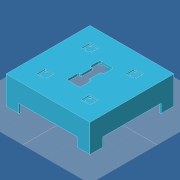
# Autodesk Inventor part: Sensorlamp_Cover
Saved by Autodesk Inventor 2016 SP2 (Build 200236200, 236)
## iProperties
Created: 2017-11-14
Part Number: Sensorlamp_Cover
Material: Generisch
Document SubType Name: Modeling
Designer: User
Density: 1 g/cm^3
Appearance: Türkis
Author: User
Autodesk Inventor part; units mm, degrees
ref_plane "YZ Plane" through (0, 0, 0) normal (1, 0, 0) x (0, 1, 0)
ref_plane "XZ Plane" through (0, 0, 0) normal (0, 1, 0) x (-1, 0, 0)
ref_plane "XY Plane" through (0, 0, 0) normal (0, 0, 1) x (1, 0, 0)
sketch "LED" plane through (0, 0, 0) normal (0, 0, 1) x (1, 0, 0)
  line L0 (-24, 24) -> (-16, 24)
  line L1 (-16, 24) -> (-16, 16)
  line L2 (-16, 16) -> (-24, 16)
  line L3 (-24, 16) -> (-24, 24)
  line L4 (-24, 24) -> (-16, 16) construction
  line L5 (-16, 24) -> (-24, 16) construction
  circle A0 centre (-22.5, 22.5) radius 1
  circle A1 centre (-17.5, 22.5) radius 1
  circle A2 centre (-22.5, 17.5) radius 1
  circle A3 centre (-17.5, 17.5) radius 1
  point P0 (-20, 20)
  point P1 (-20, 20)
  point P2 (-20, 20)
  point P3 (-20, 20)
  dimension "d11" = 8
  dimension "d12" = 8
  dimension "d20" = 2
  dimension "d21" = 5
  dimension "d22" = 5
  measures "d11" distance of L1.end L2.end
  measures "d12" distance of L0.end L1.end
  measures "d20" diameter of A0
  measures "d21" distance of A1.centre A0.centre
  measures "d22" distance of A2.centre A0.centre
sketch "Skizze1" plane through (0, 0, 0) normal (0, 0, 1) x (1, 0, 0)
  line L0 (-37.5, -37.5) -> (37.5, -37.5)
  line L1 (37.5, -37.5) -> (37.5, 37.5)
  line L2 (37.5, 37.5) -> (-37.5, 37.5)
  line L3 (-37.5, 37.5) -> (-37.5, -37.5)
  line L4 (-37.5, -37.5) -> (37.5, 37.5) construction
  line L5 (37.5, -37.5) -> (-37.5, 37.5) construction
  line L6 (-5, 15) -> (5, 15)
  line L7 (6, 14) -> (6, 6.75)
  line L8 (5, 5.75) -> (3.75, 5.75)
  line L9 (3.75, 5.75) -> (3.75, -4.25)
  line L10 (3.75, -4.25) -> (5, -4.25)
  line L11 (6, -5.25) -> (6, -14)
  line L12 (5, -15) -> (-5, -15)
  line L13 (-6, -14) -> (-6, -5.25)
  line L14 (-5, -4.25) -> (-3.75, -4.25)
  line L15 (-3.75, -4.25) -> (-3.75, 5.75)
  line L16 (-3.75, 5.75) -> (-5, 5.75)
  line L17 (-6, 6.75) -> (-6, 14)
  arc A0 (-5, 15) -> (-6, 14) centre (-5, 14) ccw
  arc A1 (6, 14) -> (5, 15) centre (5, 14) ccw
  arc A2 (-6, -14) -> (-5, -15) centre (-5, -14) ccw
  arc A3 (5, -15) -> (6, -14) centre (5, -14) ccw
  arc A4 (6, -5.25) -> (5, -4.25) centre (5, -5.25) ccw
  arc A5 (-5, -4.25) -> (-6, -5.25) centre (-5, -5.25) ccw
  arc A6 (-6, 6.75) -> (-5, 5.75) centre (-5, 6.75) ccw
  arc A7 (5, 5.75) -> (6, 6.75) centre (5, 6.75) ccw
  line L18 (0, 15) -> (0, -15) construction
  line L19 (-52.5, 0) -> (52.5, 0) projected
  line L20 (0, -52.5) -> (0, 52.5) projected
  circle A8 centre (0, -18.5) radius 3.5
  circle A9 centre (0, 18.5) radius 3.5
  line L21 (3.5, -18.5) -> (3.5, -15)
  line L22 (-3.5, -18.5) -> (-3.5, -15)
  line L23 (-3.5, 18.5) -> (-3.5, 15)
  line L24 (3.5, 18.5) -> (3.5, 15)
  circle A10 centre (0, 18.5) radius 1.25
  circle A11 centre (0, -18.5) radius 1.25
  line L25 (-24, 24) -> (-16, 24)
  line L26 (-16, 24) -> (-16, 16)
  line L27 (-16, 16) -> (-24, 16)
  line L28 (-24, 16) -> (-24, 24)
  line L29 (-24, 24) -> (-16, 16) construction
  line L30 (-16, 24) -> (-24, 16) construction
  circle A12 centre (-22.5, 22.5) radius 1
  circle A13 centre (-17.5, 22.5) radius 1
  circle A14 centre (-22.5, 17.5) radius 1
  circle A15 centre (-17.5, 17.5) radius 1
  line L31 (16, 24) -> (24, 24)
  line L32 (24, 24) -> (24, 16)
  line L33 (24, 16) -> (16, 16)
  line L34 (16, 16) -> (16, 24)
  line L35 (16, 24) -> (24, 16) construction
  line L36 (24, 24) -> (16, 16) construction
  circle A16 centre (17.5, 22.5) radius 1
  circle A17 centre (22.5, 22.5) radius 1
  circle A18 centre (17.5, 17.5) radius 1
  circle A19 centre (22.5, 17.5) radius 1
  line L37 (16, -16) -> (24, -16)
  line L38 (24, -16) -> (24, -24)
  line L39 (24, -24) -> (16, -24)
  line L40 (16, -24) -> (16, -16)
  line L41 (16, -16) -> (24, -24) construction
  line L42 (24, -16) -> (16, -24) construction
  circle A20 centre (17.5, -17.5) radius 1
  circle A21 centre (22.5, -17.5) radius 1
  circle A22 centre (17.5, -22.5) radius 1
  circle A23 centre (22.5, -22.5) radius 1
  line L43 (-24, -16) -> (-16, -16)
  line L44 (-16, -16) -> (-16, -24)
  line L45 (-16, -24) -> (-24, -24)
  line L46 (-24, -24) -> (-24, -16)
  line L47 (-24, -16) -> (-16, -24) construction
  line L48 (-16, -16) -> (-24, -24) construction
  circle A24 centre (-22.5, -17.5) radius 1
  circle A25 centre (-17.5, -17.5) radius 1
  circle A26 centre (-22.5, -22.5) radius 1
  circle A27 centre (-17.5, -22.5) radius 1
  point P0 (0, 0)
  point P1 (6, -4.25)
  point P2 (6, -15)
  point P3 (-6, -4.25)
  point P4 (-6, 5.75)
  point P5 (0, 0)
  dimension "d23" = 40
  dimension "d24" = 40
  dimension "d0" = 75
  dimension "d1" = 75
  dimension "d2" = 30
  dimension "d3" = 12
  dimension "d5" = 7.5
  dimension "d6" = 9.25
  dimension "d8" = 10.75
  dimension "d9" = 10
  dimension "d10" = 1
  dimension "d34" = 2.5
  dimension "d37" = 37
  constraints: 46 end point, 22 point on line, 21 tangent, 20 point on circle, 12 centre point, 12 perpendicular, 9 equal radius, 6 midpoint, 3 horizontal, 2 coincident, 2 collinear, 2 parallel, 1 vertical
  measures "d0" distance of L2.end L1.end
  measures "d1" distance of L1.end L0.end
  measures "d2" distance between parallel lines of L12 L6
  measures "d3" distance between parallel lines of L7 L17
  measures "d5" distance between parallel lines of L9 L15
  measures "d6" distance between parallel lines of L16 L6
  measures "d8" distance between parallel lines of L12 L14
  measures "d9" distance between parallel lines of L14 L16
  measures "d10" radius of A0
  measures "d34" diameter of A10
  measures "d37" distance of A11.centre A9.centre
extrude "Extrusion1" add sketch "Skizze1" against normal blind 2 contours L3 L19 L15 L14 A5 L13 A2 L12 L22 A8 L20 L0 | L20 A8 L21 L12 A3 L11 A4 L10 L9 L19 L1 L0 | L3 L2 L20 A9 L23 L6 A0 L17 A6 L16 L15 L19 | A8 L20 A11 | L20 A11 A8 | L19 L9 L8 A7 L7 A1 L6 L24 A9 L20 L2 L1 | A11 L20 | L20 A11 | L22 L12 A8 | A8 L12 L21 | A9 L20 A10 | L20 A10 A9 | A9 L24 L6 | L6 L23 A9 | A10 L20 | L20 A10 | L25 L26 L27 L28 | L31 L32 L33 L34 | L37 L38 L39 L40 | L43 L44 L45 L46
extrude "Extrusion2" cut sketch "Skizze1" against normal blind 1 contours L25 L26 L27 L28 | L31 L32 L33 L34 | L37 L38 L39 L40 | L43 L44 L45 L46
sketch "Skizze2" plane through (0, 0, -2) normal (0, 0, -1) x (-1, 0, 0)
  line L0 (0, -52.5) -> (0, 52.5) projected
  circle A0 centre (22.5, -17.5) radius 1 projected
  circle A1 centre (17.5, -22.5) radius 1 projected
  circle A2 centre (22.5, -22.5) radius 1 projected
  circle A3 centre (17.5, -17.5) radius 1 projected
  circle A4 centre (-17.5, -17.5) radius 1 projected
  circle A5 centre (-22.5, -22.5) radius 1 projected
  circle A6 centre (-17.5, -22.5) radius 1 projected
  circle A7 centre (-22.5, -17.5) radius 1 projected
  circle A8 centre (-17.5, 22.5) radius 1 projected
  circle A9 centre (-22.5, 17.5) radius 1 projected
  circle A10 centre (-17.5, 17.5) radius 1 projected
  circle A11 centre (-22.5, 22.5) radius 1 projected
  circle A12 centre (22.5, 22.5) radius 1 projected
  circle A13 centre (17.5, 17.5) radius 1 projected
  circle A14 centre (22.5, 17.5) radius 1 projected
  circle A15 centre (17.5, 22.5) radius 1 projected
  arc A16 (-6, 6.75) -> (-5, 5.75) centre (-5, 6.75) ccw projected
  line L1 (-6, 6.75) -> (-6, 14) projected
  arc A17 (-5, 15) -> (-6, 14) centre (-5, 14) ccw projected
  line L2 (-5, 15) -> (5, 15) projected
  arc A18 (6, 14) -> (5, 15) centre (5, 14) ccw projected
  line L3 (6, 14) -> (6, 6.75) projected
  arc A19 (5, 5.75) -> (6, 6.75) centre (5, 6.75) ccw projected
  line L4 (5, 5.75) -> (3.75, 5.75) projected
  line L5 (3.75, 5.75) -> (3.75, -4.25) projected
  line L6 (3.75, -4.25) -> (5, -4.25) projected
  arc A20 (6, -5.25) -> (5, -4.25) centre (5, -5.25) ccw projected
  line L7 (6, -5.25) -> (6, -14) projected
  arc A21 (5, -15) -> (6, -14) centre (5, -14) ccw projected
  line L8 (5, -15) -> (-5, -15) projected
  arc A22 (-6, -14) -> (-5, -15) centre (-5, -14) ccw projected
  line L9 (-6, -14) -> (-6, -5.25) projected
  arc A23 (-5, -4.25) -> (-6, -5.25) centre (-5, -5.25) ccw projected
  line L10 (-5, -4.25) -> (-3.75, -4.25) projected
  line L11 (-3.75, -4.25) -> (-3.75, 5.75) projected
  line L12 (-3.75, 5.75) -> (-5, 5.75) projected
  line L13 (-37.5, -37.5) -> (37.5, -37.5) projected
  line L14 (37.5, -37.5) -> (37.5, 37.5) projected
  line L15 (37.5, 37.5) -> (-37.5, 37.5) projected
  line L16 (-37.5, 37.5) -> (-37.5, -37.5) projected
  line L17 (52.5, 0) -> (-52.5, 0) projected
  line L18 (37.5, -26) -> (36, -26)
  line L19 (36, -26) -> (36, -36)
  line L20 (36, -36) -> (26, -36)
  line L21 (26, -36) -> (26, -37.5)
  line L22 (-37.5, -37.5) -> (37.5, -37.5) projected
  line L23 (26, -37.5) -> (37.5, -37.5)
  line L24 (37.5, -37.5) -> (37.5, -26)
  line L25 (-37.5, -26) -> (-36, -26)
  line L26 (-36, -26) -> (-36, -36)
  line L27 (-36, -36) -> (-26, -36)
  line L28 (-26, -36) -> (-26, -37.5)
  line L29 (-26, -37.5) -> (-37.5, -37.5)
  line L30 (-37.5, -37.5) -> (-37.5, -26)
  line L31 (37.5, 26) -> (36, 26)
  line L32 (36, 26) -> (36, 36)
  line L33 (36, 36) -> (26, 36)
  line L34 (26, 36) -> (26, 37.5)
  line L35 (26, 37.5) -> (37.5, 37.5)
  line L36 (37.5, 37.5) -> (37.5, 26)
  line L37 (-37.5, 26) -> (-36, 26)
  line L38 (-36, 36) -> (-26, 36)
  line L39 (-36, 26) -> (-36, 36)
  line L40 (-26, 37.5) -> (-37.5, 37.5)
  line L41 (-37.5, 37.5) -> (-37.5, 26)
  line L42 (-26, 36) -> (-26, 37.5)
  line L43 (36, -26) -> (37.5, -26)
  line L44 (37.5, -26) -> (37.5, 26)
  line L45 (37.5, 26) -> (36, 26)
  line L46 (36, 26) -> (36, -26)
  line L47 (26, 36) -> (-26, 36)
  line L48 (-26, 36) -> (-26, 37.5)
  line L49 (-26, 37.5) -> (26, 37.5)
  line L50 (26, 37.5) -> (26, 36)
  line L51 (-36, 26) -> (-37.5, 26)
  line L52 (-37.5, 26) -> (-37.5, -26)
  line L53 (-37.5, -26) -> (-36, -26)
  line L54 (-36, -26) -> (-36, 26)
  line L55 (-26, -36) -> (26, -36)
  line L56 (26, -36) -> (26, -37.5)
  line L57 (26, -37.5) -> (-26, -37.5)
  line L58 (-26, -37.5) -> (-26, -36)
  point P0 (-37.5, 37.5)
  dimension "d50" = 1.5
  dimension "d51" = 10
  constraints: 80 end point, 22 symmetric about line, 9 perpendicular, 8 parallel, 6 horizontal, 2 point on line, 1 collinear
  measures "d50" distance of L20.end L21.end
  measures "d51" distance between parallel lines of L21 L19
extrude "Extrusion3" add sketch "Skizze2" along normal blind 23 contours L13 L16 L25 L26 L27 L28 | L21 L20 L19 L18 L14 L13 | L16 L15 L42 L38 L39 L37 | L31 L32 L33 L34 L15 L14
extrude "Extrusion6" add sketch "Skizze2" along normal blind 15 contours L13 L28 L55 L0 | L0 L55 L21 L13 | L16 L17 L54 L25 | L18 L46 L17 L14 | L16 L37 L54 L17 | L17 L46 L31 L14 | L47 L42 L15 L0 | L0 L15 L34 L47
extrude "Extrusion4" add sketch "Skizze1" against normal blind 15 contours A8 L20 A11 | L20 A11 A8 | A9 L20 A10 | L20 A10 A9
equation "\"d24\" = d23"
equation "\"d1\" = d0"
